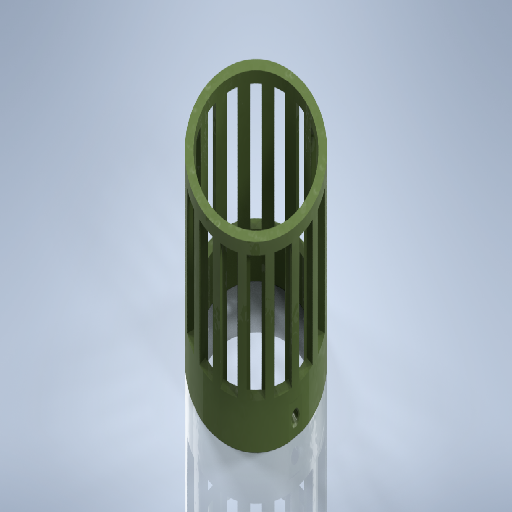
# Autodesk Inventor part: magnet_ring
Saved by Autodesk Inventor 2025 (Build 290162000, 162)
## iProperties
Created: 2026-08-03
Part Number: magnet_ring
Material: Ogólny
Document SubType Name: Modeling
Designer: zzapa
Density: 1 g/cm^3
Appearance: Ciemnooliwkowa
Author: zzapa
Autodesk Inventor part; units mm, degrees
ref_plane "YZ Plane" through (0, 0, 0) normal (1, 0, 0) x (0, 1, 0)
ref_plane "XZ Plane" through (0, 0, 0) normal (0, 1, 0) x (-1, 0, 0)
sketch "Szkic1" plane through (0, 0, 0) normal (0, 0, 1) x (1, 0, 0)
  line L0 (26.95, 18) -> (23.65, 18)
  line L1 (23.65, 18) -> (23.65, -18)
  line L2 (23.65, -18) -> (26.95, -18)
  line L3 (26.95, -18) -> (26.95, 18)
  line L4 (-5.39, 0) -> (32.34, 0) projected
  line L5 (0, -25.2) -> (0, 25.2) projected
  point P0 (0, 0)
  point P1 (23.65, 0)
  dimension "d0" = 26.95
  dimension "d1" = 3.3
  dimension "d15" = 36
  constraints: 8 end point, 2 parallel, 1 horizontal, 1 midpoint, 1 perpendicular, 1 point on line
  measures "d0" distance from line of point (0, 0) L3
  measures "d1" distance of L0.start L0.end
  measures "d15" distance of L2.end L0.start
revolve "Obrót1" add sketch "Szkic1" angle 360 about axis through (0, -10, 0) along (0, 1, 0)
sketch "Szkic2" plane through (0, 0, 0) normal (0, 1, 0) x (-1, 0, 0)
  line L0 (23.615164, -3.55) -> (26.715164, -3.55)
  line L1 (26.715164, -3.55) -> (26.715164, 3.55)
  line L2 (26.715164, 3.55) -> (23.615164, 3.55)
  line L3 (23.615164, 3.55) -> (23.615164, -3.55)
  circle A0 centre (0, 0) radius 26.95
  line L4 (37.73, 0) -> (-37.73, 0)
  line L5 (26.715164, -3.55) -> (26.95, -3.55)
  line L6 (26.95, -3.55) -> (26.95, 3.55)
  line L7 (26.95, 3.55) -> (26.715164, 3.55)
  line L8 (26.715164, 3.55) -> (26.715164, -3.55)
  line L9 (23.55207, -2.15) -> (23.615164, -2.15)
  line L10 (23.615164, -2.15) -> (23.615164, 2.15)
  line L11 (23.615164, 2.15) -> (23.55207, 2.15)
  line L12 (23.55207, 2.15) -> (23.55207, -2.15)
  circle A1 centre (0, 0) radius 23.65
  line L13 (22.582045, 7.026646) -> (22.640336, 7.050791)
  line L14 (20.936506, 10.999328) -> (22.582045, 7.026646)
  line L15 (22.640336, 7.050791) -> (20.994798, 11.023473)
  line L16 (20.459041, 12.316904) -> (23.176093, 5.75736)
  line L17 (23.176093, 5.75736) -> (26.04012, 6.943678)
  line L18 (23.323067, 13.503223) -> (20.459041, 12.316904)
  line L19 (26.04012, 6.943678) -> (26.25708, 7.033546)
  line L20 (23.540027, 13.593091) -> (23.323067, 13.503223)
  line L21 (26.04012, 6.943678) -> (23.323067, 13.503223)
  line L22 (23.323067, 13.503223) -> (26.04012, 6.943678)
  line L23 (26.25708, 7.033546) -> (23.540027, 13.593091)
  line L24 (20.994798, 11.023473) -> (20.936506, 10.999328)
  line L25 (18.174108, 15.133549) -> (18.218722, 15.178163)
  line L26 (15.133549, 18.174108) -> (18.174108, 15.133549)
  line L27 (18.218722, 15.178163) -> (15.178163, 18.218722)
  line L28 (14.188214, 19.208672) -> (19.208672, 14.188214)
  line L29 (19.208672, 14.188214) -> (21.400703, 16.380245)
  line L30 (16.380245, 21.400703) -> (14.188214, 19.208672)
  line L31 (21.400703, 16.380245) -> (21.566757, 16.546299)
  line L32 (16.546299, 21.566757) -> (16.380245, 21.400703)
  line L33 (21.400703, 16.380245) -> (16.380245, 21.400703)
  line L34 (16.380245, 21.400703) -> (21.400703, 16.380245)
  line L35 (21.566757, 16.546299) -> (16.546299, 21.566757)
  line L36 (15.178163, 18.218722) -> (15.133549, 18.174108)
  line L37 (10.999328, 20.936506) -> (11.023473, 20.994798)
  line L38 (7.026646, 22.582045) -> (10.999328, 20.936506)
  line L39 (11.023473, 20.994798) -> (7.050791, 22.640336)
  line L40 (5.75736, 23.176093) -> (12.316904, 20.459041)
  line L41 (12.316904, 20.459041) -> (13.503223, 23.323067)
  line L42 (6.943678, 26.04012) -> (5.75736, 23.176093)
  line L43 (13.503223, 23.323067) -> (13.593091, 23.540027)
  line L44 (7.033546, 26.25708) -> (6.943678, 26.04012)
  line L45 (13.503223, 23.323067) -> (6.943678, 26.04012)
  line L46 (6.943678, 26.04012) -> (13.503223, 23.323067)
  line L47 (13.593091, 23.540027) -> (7.033546, 26.25708)
  line L48 (7.050791, 22.640336) -> (7.026646, 22.582045)
  line L49 (2.15, 23.55207) -> (2.15, 23.615164)
  line L50 (-2.15, 23.55207) -> (2.15, 23.55207)
  line L51 (2.15, 23.615164) -> (-2.15, 23.615164)
  line L52 (-3.55, 23.615164) -> (3.55, 23.615164)
  line L53 (3.55, 23.615164) -> (3.55, 26.715164)
  line L54 (-3.55, 26.715164) -> (-3.55, 23.615164)
  line L55 (3.55, 26.715164) -> (3.55, 26.95)
  line L56 (-3.55, 26.95) -> (-3.55, 26.715164)
  line L57 (3.55, 26.715164) -> (-3.55, 26.715164)
  line L58 (-3.55, 26.715164) -> (3.55, 26.715164)
  line L59 (3.55, 26.95) -> (-3.55, 26.95)
  line L60 (-2.15, 23.615164) -> (-2.15, 23.55207)
  line L61 (-7.026646, 22.582045) -> (-7.050791, 22.640336)
  line L62 (-10.999328, 20.936506) -> (-7.026646, 22.582045)
  line L63 (-7.050791, 22.640336) -> (-11.023473, 20.994798)
  line L64 (-12.316904, 20.459041) -> (-5.75736, 23.176093)
  line L65 (-5.75736, 23.176093) -> (-6.943678, 26.04012)
  line L66 (-13.503223, 23.323067) -> (-12.316904, 20.459041)
  line L67 (-6.943678, 26.04012) -> (-7.033546, 26.25708)
  line L68 (-13.593091, 23.540027) -> (-13.503223, 23.323067)
  line L69 (-6.943678, 26.04012) -> (-13.503223, 23.323067)
  line L70 (-13.503223, 23.323067) -> (-6.943678, 26.04012)
  line L71 (-7.033546, 26.25708) -> (-13.593091, 23.540027)
  line L72 (-11.023473, 20.994798) -> (-10.999328, 20.936506)
  line L73 (-15.133549, 18.174108) -> (-15.178163, 18.218722)
  line L74 (-18.174108, 15.133549) -> (-15.133549, 18.174108)
  line L75 (-15.178163, 18.218722) -> (-18.218722, 15.178163)
  line L76 (-19.208672, 14.188214) -> (-14.188214, 19.208672)
  line L77 (-14.188214, 19.208672) -> (-16.380245, 21.400703)
  line L78 (-21.400703, 16.380245) -> (-19.208672, 14.188214)
  line L79 (-16.380245, 21.400703) -> (-16.546299, 21.566757)
  line L80 (-21.566757, 16.546299) -> (-21.400703, 16.380245)
  line L81 (-16.380245, 21.400703) -> (-21.400703, 16.380245)
  line L82 (-21.400703, 16.380245) -> (-16.380245, 21.400703)
  line L83 (-16.546299, 21.566757) -> (-21.566757, 16.546299)
  line L84 (-18.218722, 15.178163) -> (-18.174108, 15.133549)
  line L85 (-20.936506, 10.999328) -> (-20.994798, 11.023473)
  line L86 (-22.582045, 7.026646) -> (-20.936506, 10.999328)
  line L87 (-20.994798, 11.023473) -> (-22.640336, 7.050791)
  line L88 (-23.176093, 5.75736) -> (-20.459041, 12.316904)
  line L89 (-20.459041, 12.316904) -> (-23.323067, 13.503223)
  line L90 (-26.04012, 6.943678) -> (-23.176093, 5.75736)
  line L91 (-23.323067, 13.503223) -> (-23.540027, 13.593091)
  line L92 (-26.25708, 7.033546) -> (-26.04012, 6.943678)
  line L93 (-23.323067, 13.503223) -> (-26.04012, 6.943678)
  line L94 (-26.04012, 6.943678) -> (-23.323067, 13.503223)
  line L95 (-23.540027, 13.593091) -> (-26.25708, 7.033546)
  line L96 (-22.640336, 7.050791) -> (-22.582045, 7.026646)
  line L97 (-23.55207, 2.15) -> (-23.615164, 2.15)
  line L98 (-23.55207, -2.15) -> (-23.55207, 2.15)
  line L99 (-23.615164, 2.15) -> (-23.615164, -2.15)
  line L100 (-23.615164, -3.55) -> (-23.615164, 3.55)
  line L101 (-23.615164, 3.55) -> (-26.715164, 3.55)
  line L102 (-26.715164, -3.55) -> (-23.615164, -3.55)
  line L103 (-26.715164, 3.55) -> (-26.95, 3.55)
  line L104 (-26.95, -3.55) -> (-26.715164, -3.55)
  line L105 (-26.715164, 3.55) -> (-26.715164, -3.55)
  line L106 (-26.715164, -3.55) -> (-26.715164, 3.55)
  line L107 (-26.95, 3.55) -> (-26.95, -3.55)
  line L108 (-23.615164, -2.15) -> (-23.55207, -2.15)
  line L109 (-22.582045, -7.026646) -> (-22.640336, -7.050791)
  line L110 (-20.936506, -10.999328) -> (-22.582045, -7.026646)
  line L111 (-22.640336, -7.050791) -> (-20.994798, -11.023473)
  line L112 (-20.459041, -12.316904) -> (-23.176093, -5.75736)
  line L113 (-23.176093, -5.75736) -> (-26.04012, -6.943678)
  line L114 (-23.323067, -13.503223) -> (-20.459041, -12.316904)
  line L115 (-26.04012, -6.943678) -> (-26.25708, -7.033546)
  line L116 (-23.540027, -13.593091) -> (-23.323067, -13.503223)
  line L117 (-26.04012, -6.943678) -> (-23.323067, -13.503223)
  line L118 (-23.323067, -13.503223) -> (-26.04012, -6.943678)
  line L119 (-26.25708, -7.033546) -> (-23.540027, -13.593091)
  line L120 (-20.994798, -11.023473) -> (-20.936506, -10.999328)
  line L121 (-18.174108, -15.133549) -> (-18.218722, -15.178163)
  line L122 (-15.133549, -18.174108) -> (-18.174108, -15.133549)
  line L123 (-18.218722, -15.178163) -> (-15.178163, -18.218722)
  line L124 (-14.188214, -19.208672) -> (-19.208672, -14.188214)
  line L125 (-19.208672, -14.188214) -> (-21.400703, -16.380245)
  line L126 (-16.380245, -21.400703) -> (-14.188214, -19.208672)
  line L127 (-21.400703, -16.380245) -> (-21.566757, -16.546299)
  line L128 (-16.546299, -21.566757) -> (-16.380245, -21.400703)
  line L129 (-21.400703, -16.380245) -> (-16.380245, -21.400703)
  line L130 (-16.380245, -21.400703) -> (-21.400703, -16.380245)
  line L131 (-21.566757, -16.546299) -> (-16.546299, -21.566757)
  line L132 (-15.178163, -18.218722) -> (-15.133549, -18.174108)
  line L133 (-10.999328, -20.936506) -> (-11.023473, -20.994798)
  line L134 (-7.026646, -22.582045) -> (-10.999328, -20.936506)
  line L135 (-11.023473, -20.994798) -> (-7.050791, -22.640336)
  line L136 (-5.75736, -23.176093) -> (-12.316904, -20.459041)
  line L137 (-12.316904, -20.459041) -> (-13.503223, -23.323067)
  line L138 (-6.943678, -26.04012) -> (-5.75736, -23.176093)
  line L139 (-13.503223, -23.323067) -> (-13.593091, -23.540027)
  line L140 (-7.033546, -26.25708) -> (-6.943678, -26.04012)
  line L141 (-13.503223, -23.323067) -> (-6.943678, -26.04012)
  line L142 (-6.943678, -26.04012) -> (-13.503223, -23.323067)
  line L143 (-13.593091, -23.540027) -> (-7.033546, -26.25708)
  line L144 (-7.050791, -22.640336) -> (-7.026646, -22.582045)
  line L145 (-2.15, -23.55207) -> (-2.15, -23.615164)
  line L146 (2.15, -23.55207) -> (-2.15, -23.55207)
  line L147 (-2.15, -23.615164) -> (2.15, -23.615164)
  line L148 (3.55, -23.615164) -> (-3.55, -23.615164)
  line L149 (-3.55, -23.615164) -> (-3.55, -26.715164)
  line L150 (3.55, -26.715164) -> (3.55, -23.615164)
  line L151 (-3.55, -26.715164) -> (-3.55, -26.95)
  line L152 (3.55, -26.95) -> (3.55, -26.715164)
  line L153 (-3.55, -26.715164) -> (3.55, -26.715164)
  line L154 (3.55, -26.715164) -> (-3.55, -26.715164)
  line L155 (-3.55, -26.95) -> (3.55, -26.95)
  line L156 (2.15, -23.615164) -> (2.15, -23.55207)
  line L157 (7.026646, -22.582045) -> (7.050791, -22.640336)
  line L158 (10.999328, -20.936506) -> (7.026646, -22.582045)
  line L159 (7.050791, -22.640336) -> (11.023473, -20.994798)
  line L160 (12.316904, -20.459041) -> (5.75736, -23.176093)
  line L161 (5.75736, -23.176093) -> (6.943678, -26.04012)
  line L162 (13.503223, -23.323067) -> (12.316904, -20.459041)
  line L163 (6.943678, -26.04012) -> (7.033546, -26.25708)
  line L164 (13.593091, -23.540027) -> (13.503223, -23.323067)
  line L165 (6.943678, -26.04012) -> (13.503223, -23.323067)
  line L166 (13.503223, -23.323067) -> (6.943678, -26.04012)
  line L167 (7.033546, -26.25708) -> (13.593091, -23.540027)
  line L168 (11.023473, -20.994798) -> (10.999328, -20.936506)
  line L169 (15.133549, -18.174108) -> (15.178163, -18.218722)
  line L170 (18.174108, -15.133549) -> (15.133549, -18.174108)
  line L171 (15.178163, -18.218722) -> (18.218722, -15.178163)
  line L172 (19.208672, -14.188214) -> (14.188214, -19.208672)
  line L173 (14.188214, -19.208672) -> (16.380245, -21.400703)
  line L174 (21.400703, -16.380245) -> (19.208672, -14.188214)
  line L175 (16.380245, -21.400703) -> (16.546299, -21.566757)
  line L176 (21.566757, -16.546299) -> (21.400703, -16.380245)
  line L177 (16.380245, -21.400703) -> (21.400703, -16.380245)
  line L178 (21.400703, -16.380245) -> (16.380245, -21.400703)
  line L179 (16.546299, -21.566757) -> (21.566757, -16.546299)
  line L180 (18.218722, -15.178163) -> (18.174108, -15.133549)
  line L181 (20.936506, -10.999328) -> (20.994798, -11.023473)
  line L182 (22.582045, -7.026646) -> (20.936506, -10.999328)
  line L183 (20.994798, -11.023473) -> (22.640336, -7.050791)
  line L184 (23.176093, -5.75736) -> (20.459041, -12.316904)
  line L185 (20.459041, -12.316904) -> (23.323067, -13.503223)
  line L186 (26.04012, -6.943678) -> (23.176093, -5.75736)
  line L187 (23.323067, -13.503223) -> (23.540027, -13.593091)
  line L188 (26.25708, -7.033546) -> (26.04012, -6.943678)
  line L189 (23.323067, -13.503223) -> (26.04012, -6.943678)
  line L190 (26.04012, -6.943678) -> (23.323067, -13.503223)
  line L191 (23.540027, -13.593091) -> (26.25708, -7.033546)
  line L192 (22.640336, -7.050791) -> (22.582045, -7.026646)
  point P0 (26.715164, 0)
  point P1 (26.95, 0)
  point P2 (23.55207, 0)
  point P3 (21.759275, 9.012987)
  point P4 (24.681593, 10.223451)
  point P5 (24.898553, 10.313319)
  point P6 (16.653828, 16.653828)
  point P7 (18.890474, 18.890474)
  point P8 (19.056528, 19.056528)
  point P9 (9.012987, 21.759275)
  point P10 (10.223451, 24.681593)
  point P11 (10.313319, 24.898553)
  point P12 (0, 23.55207)
  point P13 (0, 26.715164)
  point P14 (0, 26.95)
  point P15 (-9.012987, 21.759275)
  point P16 (-10.223451, 24.681593)
  point P17 (-10.313319, 24.898553)
  point P18 (-16.653828, 16.653828)
  point P19 (-18.890474, 18.890474)
  point P20 (-19.056528, 19.056528)
  point P21 (-21.759275, 9.012987)
  point P22 (-24.681593, 10.223451)
  point P23 (-24.898553, 10.313319)
  point P24 (-23.55207, 0)
  point P25 (-26.715164, 0)
  point P26 (-26.95, 0)
  point P27 (-21.759275, -9.012987)
  point P28 (-24.681593, -10.223451)
  point P29 (-24.898553, -10.313319)
  point P30 (-16.653828, -16.653828)
  point P31 (-18.890474, -18.890474)
  point P32 (-19.056528, -19.056528)
  point P33 (-9.012987, -21.759275)
  point P34 (-10.223451, -24.681593)
  point P35 (-10.313319, -24.898553)
  point P36 (0, -23.55207)
  point P37 (0, -26.715164)
  point P38 (0, -26.95)
  point P39 (9.012987, -21.759275)
  point P40 (10.223451, -24.681593)
  point P41 (10.313319, -24.898553)
  point P42 (16.653828, -16.653828)
  point P43 (18.890474, -18.890474)
  point P44 (19.056528, -19.056528)
  point P45 (21.759275, -9.012987)
  point P46 (24.681593, -10.223451)
  point P47 (24.898553, -10.313319)
  point P48 (22.582045, 7.026646)
  point P49 (22.640336, 7.050791)
  point P50 (20.994798, 11.023473)
  point P51 (20.936506, 10.999328)
  point P52 (18.174108, 15.133549)
  point P53 (18.218722, 15.178163)
  point P54 (15.178163, 18.218722)
  point P55 (15.133549, 18.174108)
  point P56 (10.999328, 20.936506)
  point P57 (11.023473, 20.994798)
  point P58 (7.050791, 22.640336)
  point P59 (2.15, 23.55207)
  point P60 (2.15, 23.615164)
  point P61 (-2.15, 23.615164)
  point P62 (-7.026646, 22.582045)
  point P63 (-7.050791, 22.640336)
  point P64 (-11.023473, 20.994798)
  point P65 (-10.999328, 20.936506)
  point P66 (-15.133549, 18.174108)
  point P67 (-15.178163, 18.218722)
  point P68 (-18.218722, 15.178163)
  point P69 (-18.174108, 15.133549)
  point P70 (-20.936506, 10.999328)
  point P71 (-20.994798, 11.023473)
  point P72 (-22.640336, 7.050791)
  point P73 (-23.55207, 2.15)
  point P74 (-23.615164, 2.15)
  point P75 (-23.615164, -2.15)
  point P76 (-23.55207, -2.15)
  point P77 (-22.582045, -7.026646)
  point P78 (-22.640336, -7.050791)
  point P79 (-20.994798, -11.023473)
  point P80 (-20.936506, -10.999328)
  point P81 (-18.174108, -15.133549)
  point P82 (-18.218722, -15.178163)
  point P83 (-15.178163, -18.218722)
  point P84 (-15.133549, -18.174108)
  point P85 (-10.999328, -20.936506)
  point P86 (-11.023473, -20.994798)
  point P87 (-7.050791, -22.640336)
  point P88 (-2.15, -23.55207)
  point P89 (-2.15, -23.615164)
  point P90 (2.15, -23.615164)
  point P91 (2.15, -23.55207)
  point P92 (7.026646, -22.582045)
  point P93 (11.023473, -20.994798)
  point P94 (10.999328, -20.936506)
  point P95 (15.133549, -18.174108)
  point P96 (18.218722, -15.178163)
  point P97 (18.174108, -15.133549)
  point P98 (20.936506, -10.999328)
  point P99 (22.640336, -7.050791)
  point P100 (22.582045, -7.026646)
  point P101 (23.615164, -2.15)
  point P102 (23.615164, 2.15)
  dimension "d3" = 7.1
  dimension "d4" = 3.1
  dimension "d16" = 1.4
  dimension "d19" = 360
  constraints: 384 end point, 6 parallel, 3 horizontal, 3 midpoint, 3 perpendicular, 2 collinear, 2 point on circle, 2 point on line, 419 other
  measures "d3" distance of L0.end L1.end
  measures "d4" distance of L1.end L2.end
  measures "d16" distance between parallel lines of L11 L2
extrude "Pocket" cut sketch "Szkic2" along normal mid plane 30.3 contours L3 A1 L4 L1 L0 | L1 L4 A0 | A0 L6 L5 | L9 A1 L3 | L4 A1 L3 L2 L1 | L1 A0 L4 | L188 L191 A0 | L189 L185 L184 L183 A1 L186 | A0 L189 | A0 L7 L6 | A1 L12 L4 L3 | L3 L4 A1 | A1 L182 L170 L158 L146 L134 L122 L110 L98 L4 L12 | L4 L3 A1 | L191 L187 A0 | L4 L12 A1 L3 | L4 L98 A1 L86 L74 L62 L50 L38 L26 L14 L12 | L192 L183 A1 | A1 L183 L182 | L21 A0 | A0 L23 L19 | L17 L16 L15 A1 L18 L21 | A1 L11 L3 | L176 L179 A0 | L177 L173 L172 L171 A1 L174 | A0 L177 | L98 A1 L99 L4 | L4 L99 A1 L98 | A1 L183 | A1 L183 L181 | A0 L20 L23 | L179 L175 A0 | L99 A1 L4 | L4 A1 L99 | L108 L99 A1 | A1 L99 L97 | L14 A1 L15 | A1 L15 L13 | L180 L171 A1 | A1 L171 L170 | L33 A0 | A0 L35 L31 | L29 L28 L27 A1 L30 L33 | L164 L167 A0 | L165 L161 L160 L159 A1 L162 | A0 L165 | A1 L99 L100 L102 A0 L4 | L4 A0 L101 L100 L99 A1 | L110 A1 L111 | A1 L111 L109 | L96 L87 A1 | A1 L87 L86 | L15 A1 | L24 L15 A1 | A1 L171 | A1 L171 L169 | A0 L32 L35 | L167 L163 A0 | L111 A1 | A1 L111 L112 L114 L117 L113 | L120 L111 A1 | L87 L88 L90 L93 L89 A1 | A1 L87 | A1 L87 L85 | L26 A1 L27 | A1 L27 L25 | L168 L159 A1 | A1 L159 L158 | L45 A0 | A0 L47 L43 | L41 L40 L39 A1 L42 L45 | L152 L155 A0 | L153 L149 L148 L147 A1 L150 | A0 L153 | L122 A1 L123 | A1 L123 L121 | L84 L75 A1 | A1 L75 L74 | L27 A1 | L36 L27 A1 | A1 L159 | A1 L159 L157 | A0 L44 L47 | L155 L151 A0 | L92 L95 A0 | A0 L93 | L117 A0 | A0 L119 L115 | L123 A1 | A1 L123 L124 L126 L129 L125 | L132 L123 A1 | L75 L76 L78 L81 L77 A1 | A1 L75 | A1 L75 L73 | L38 A1 L39 | A1 L39 L37 | L156 L147 A1 | A1 L147 L146 | L57 A0 | A0 L59 L55 | L53 L52 L51 A1 L54 L57 | L140 L143 A0 | L141 L137 L136 L135 A1 L138 | A0 L141 | L95 L91 A0 | A0 L116 L119 | L134 A1 L135 | A1 L135 L133 | L72 L63 A1 | A1 L63 L62 | L39 A1 | L48 L39 A1 | A1 L147 | A1 L147 L145 | A0 L56 L59 | L143 L139 A0 | L80 L83 A0 | A0 L81 | L129 A0 | A0 L131 L127 | L135 A1 | L144 L135 A1 | L63 L64 L66 L69 L65 A1 | A1 L63 | A1 L63 L61 | L50 A1 L51 | A1 L51 L49 | L69 A0 | A0 L71 L67 | L128 L131 A0 | L83 L79 A0 | L60 L51 A1 | L51 A1 | A0 L68 L71
sketch "Szkic3" plane through (0, -18, 0) normal (0, -1, 0) x (1, 0, 0)
  circle A0 centre (0, 0) radius 26.95
  circle A1 centre (0, 0) radius 23.65
  circle A2 centre (0, 0) radius 23.65
  line L0 (3.55, -26.715164) -> (3.55, -23.615164)
  circle A3 centre (0, 0) radius 26.95
  constraints: 2 coincident, 1 centre point, 1 concentric, 4 other
extrude "Wyciągnięcie proste2" add sketch "Szkic3" along normal blind 8
ref_plane "Płaszczyzna konstrukcyjna3" through (-26.432163, 0, -5.257684) normal (-0.9807853, 0, -0.1950903) x (0, -1, 0)
ref_plane "Płaszczyzna konstrukcyjna2" through (-4.697348, -15.15, 23.615164) normal (-0.9807853, 0, -0.1950903) x (0, -1, 0)
sketch "Szkic5" plane through (0, -26, 0) normal (0, -1, 0) x (1, 0, 0)
  circle A0 centre (0, 0) radius 26.95
  line L0 (-17.686376, -49.225728) -> (-35.630211, 40.984024)
  line L1 (-27.021778, -2.293489) -> (-25.842548, -8.22188)
  line L2 (-25.842548, -8.22188) -> (-25.675815, -8.188714)
  line L3 (-25.675815, -8.188714) -> (-26.855045, -2.260323)
  line L4 (-26.855045, -2.260323) -> (-27.021778, -2.293489)
  line L5 (0, 0) -> (-38.832746, -7.724313)
  point P0 (-26.432163, -5.257684)
  dimension "d30" = 0.17
  constraints: 10 end point, 3 point on line, 2 parallel, 2 perpendicular, 1 midpoint, 2 other
  measures "d30" distance between parallel lines of L0 L3
sketch "Szkic5 outline for Wyciągnięcie proste4" plane through (0, -26, 0) normal (0, -1, 0) x (1, 0, 0)
  line L0 (-25.675815, -8.188714) -> (-26.855045, -2.260323)
  line L1 (-25.842548, -8.22188) -> (-25.675815, -8.188714)
  line L2 (-27.021778, -2.293489) -> (-25.842548, -8.22188)
  line L3 (-26.855045, -2.260323) -> (-27.021778, -2.293489)
extrude "Wyciągnięcie proste4" cut sketch "Szkic5 outline for Wyciągnięcie proste4" against normal blind 8
mirror "Odbij1" about plane through (-4.697348, -15.15, 23.615164) normal (-0.9807853, 0, -0.1950903) of "Wyciągnięcie proste4"
sketch "Szkic6" plane through (-26.855045, -26, -2.260323) normal (-0.9807853, 0, -0.1950903) x (-0.1950903, 0, 0.9807853)
  line L0 (0, 8) -> (-6.044535, 8)
  line L1 (0, 0) -> (-6.044535, 0)
  line L2 (-3.022267, 8) -> (-3.022267, 0)
  line L3 (20.627733, 0) -> (-26.672267, 0)
  point P0 (-3.022267, 26)
  point P1 (-3.022267, 4)
  dimension "d31" = 4
  constraints: 3 midpoint, 2 end point
  measures "d31" distance from line of L1 point (-3.022, 4)
hole "Otwór1" at (-26.26543, -22, -5.224519) direction (0.9807853, 0, 0.1950903) diameter 2.9 end through all
chamfer "Faza1" distance 0.5 angle 45 2 edges at (-25.9825, -22, -6.6467) (26.5483, -22, 3.8024)
sketch "Szkic7" plane through (-26.855045, -26, -2.260323) normal (-0.9807853, 0, -0.1950903) x (-0.1950903, 0, 0.9807853)
  circle A0 centre (-3.022267, 4) radius 1.45
  line L0 (-3.022267, 4) -> (-3.022267, 8)
  line L1 (0, 0) -> (-6.044535, 0)
  line L2 (0, 8) -> (-6.044535, 8)
  line L3 (-3.022267, 5.674316) -> (-3.747267, 5.255737)
  line L4 (-3.022267, 5.674316) -> (-2.297267, 5.255737)
  point P0 (-3.022267, 26)
  point P1 (-2.297267, 5.255737)
  dimension "d45" = 120
  constraints: 6 end point, 1 midpoint, 1 point on line, 1 symmetric about line, 1 vertical, 3 other
  measures "d45" angle of L3 L4
extrude "Wyciągnięcie proste5" cut sketch "Szkic7" against normal through all contours A0 L0 L4 | L3 L0 A0
equation "\"d0\" = magnet_ring_r"
equation "\"d1\" = magnet_ring_d"
equation "\"d15\" = magnet_ring_h"
equation "\"d3\" = magnet_ring_pocket_mag_size_x"
equation "\"d4\" = magnet_ring_pocket_mag_size_y"
equation "\"d16\" = magnet_ring_pocket_radial_cut"
equation "\"d9\" = 3 * magnet_ring_pocket_mag_size_z"
equation "\"d21\" = magnet_ring_insert_part_lengthen"
equation "\"d30\" = magnet_ring_insert_part_axial_flat_cut"
equation "\"d31\" = magnet_ring_insert_pos"
equation "\"d32\" = insert_m2_d"
equation "\"d42\" = insert_m2_corner"
equation "\"stator_r_out\" = 30.15"
equation "\"stator_out_d\" = 3.2"
equation "\"stator_h\" = 45"
equation "\"mag_size_x\" = 7"
equation "\"mag_size_y\" = 3"
equation "\"mag_corner_r\" = 0.4"
equation "\"magnet_ring_r\" = 26.95"
equation "\"magnet_ring_d\" = 3.3"
equation "\"magnet_ring_pocket_mag_size_y\" = 3.1"
equation "\"magnet_ring_pocket_mag_size_x\" = 7.1"
equation "\"magnet_ring_pocket_mag_size_z\" = 10.1"
equation "\"magnet_ring_mag_count\" = 16"
equation "\"magnet_ring_h\" = 36"
equation "\"magnet_ring_pocket_radial_cut\" = 1.4"
equation "\"casing_d\" = 3"
equation "\"casing_r_in\" = 30.15"
equation "\"rotor_core_r\" = 14.97"
equation "\"coil_groove_ang\" = 18"
equation "\"rotor_out_r\" = 22.5"
equation "\"rotor_coil_groove_in_r\" = 17"
equation "\"rotor_coil_groove_ang\" = 18deg"
equation "\"rotor_coil_groove_in_correction_r\" = 18"
equation "\"rotor_plastic_h\" = 32"
equation "\"rotor_teeth_d\" = 1.5"
equation "\"shaft_d\" = 8"
equation "\"insert25m_d\" = 2.9"
equation "\"insert25m_corner\" = 0.5"
equation "\"insert25m_h\" = 7"
equation "\"rotor_plastic_insert_r\" = 37"
equation "\"shaft_lock_1_d\" = 8.1"
equation "\"shaf_lock_1_D\" = 32"
equation "\"shaft_lock_1_D\" = 44"
equation "\"shaft_lock_1_h1\" = 3.5"
equation "\"shaft_lock_1_insert_part_h\" = 8"
equation "\"shaft_lock_1_corner\" = 2"
equation "\"shaft_lock_1_insert_part_a\" = 18"
equation "\"shaft_lock_2_h1\" = 3.5"
equation "\"shaft_lock_2_d\" = 8.1"
equation "\"shaft_lock_2_insert_part_a\" = 18"
equation "\"shaft_lock_2_D\" = 44"
equation "\"shaft_lock_2_corner\" = 2"
equation "\"shaft_lock_2_insert_part_h\" = 7"
equation "\"shaft_lock_2_rotor_insert_grove_d_in\" = 36"
equation "\"shaft_lock_2_rotor_insert_grove_width_out\" = 5.5"
equation "\"shaft_lock_2_rotor_insert_grove_width_in\" = 7.6"
equation "\"shaft_lock_2_rotor_insert_r\" = 37"
equation "\"shaft_lock_2_rotor_insert_screw_d\" = 2.6"
equation "\"insert25m_pocket_d\" = 2.6"
equation "\"insert25m_pocket_D\" = 4.5"
equation "\"insert25m_pocket_nut_h\" = 1.5"
equation "\"insert_m2_pocket_d\" = 2.6"
equation "\"insert_m2_h\" = 7"
equation "\"insert_m2_d\" = 2.9"
equation "\"insert_m2_corner\" = 0.5"
equation "\"insert_m2_pocket_D\" = 4.5"
equation "\"insert_m2_pocket_nut_h\" = 1.5"
equation "\"shaft_lock_1_insert_part_corner\" = 6"
equation "\"shaft_lock_1_insert_part_pos\" = 4"
equation "\"shaft_lock_1_rotor_insert_grove_width_in\" = 7.6"
equation "\"shaft_lock_1_rotor_insert_r\" = 37"
equation "\"shaft_lock_1_rotor_insert_grove_d_in\" = 36"
equation "\"shaft_lock_1_rotor_insert_grove_width_out\" = 5.5"
equation "\"shaft_lock_1_shaft_insert_axial_cut_out_width\" = 12"
equation "\"shaft_lock_1_shaft_insert_axial_cut_in_width\" = 5.4"
equation "\"shaft_lock_1_shaft_insert_corner\" = 2"
equation "\"shaft_lock_1_shaft_insert_corner_finish\" = 0.5"
equation "\"shaft_lock_1_shaft_insert_pos\" = 2.5"
equation "\"shaft_lock_2_shaft_insert_corner\" = 2"
equation "\"shaft_lock_2_shaft_insert_pos\" = 2.5"
equation "\"shaft_lock_2_shaft_insert_axial_cut_in_width\" = 5.4"
equation "\"shaft_lock_2_shaft_insert_axial_cut_out_width\" = 12"
equation "\"shaft_lock_2_shaft_insert_corner_finish\" = 0.5"
equation "\"commutator_plate_D\" = 22"
equation "\"commutator_plastic_d\" = 1"
equation "\"commutator_plastic_h\" = 17"
equation "\"commutator_plate_ang\" = 55deg"
equation "\"commutator_plate_d\" = 1"
equation "\"commutator_plate_h\" = 17"
equation "\"commutator_plastic_shaft_d\" = 8.1"
equation "\"commutator_plastic_insert_cut_deepness\" = 0.5"
equation "\"commutator_plastic_insert_cut_length\" = 6"
equation "\"commutator_plastic_insert_pos\" = 3"
equation "\"commutator_plate_insert_pos\" = 3"
equation "\"casing_lock_hole_r\" = 14.25"
equation "\"casing_lock_h\" = 8"
equation "\"casing_stator_fix_r\" = 23"
equation "\"casing_stator_fix_h\" = 6"
equation "\"magnet_ring_insert_part_lengthen\" = 8"
equation "\"casing_sidebar_length\" = 3"
equation "\"casing_vent_hole_length\" = 4"
equation "\"casing_vent_hole_width\" = 6"
equation "\"sleeve_cup_r\" = 22"
equation "\"sleeve_cup_h\" = 4.5"
equation "\"sleeve_h\" = 7"
equation "\"sleeve_d\" = 3"
equation "\"sleeve_in_r\" = 11.1"
equation "\"casing_head_insert_r\" = 19"
equation "\"sleeve_head_insert_r\" = 19"
equation "\"magnet_ring_insert_part_radius_cut\" = 0.17"
equation "\"magnet_ring_insert_part_axial_flat_cut\" = 0.17"
equation "\"magnet_ring_insert_pos\" = 4"
equation "\"casing_radial_stator_insert_pos\" = 18.1"
equation "\"stator_radial_screw_d\" = 4"
equation "\"stator_radial_screw_pos\" = 4"
equation "\"rotor_sleeve_out_D\" = 10.5"
equation "\"rotor_sleeve_in_D\" = 8.15"
equation "\"rotor_sleeve_h\" = 32"
equation "\"carbon_brush_batt_h\" = 8"
equation "\"carbon_brush_batt_d\" = 4"
equation "\"brush_cart_outer_holder_width\" = 5.5"
equation "\"brush_cart_outer_holder_arc_r\" = 33.15"
equation "\"brush_cart_outer_holder_arc_pos\" = 1.5"
equation "\"casing_cart_hole_corner\" = 1"
equation "\"casing_cart_hole_width\" = 2.6"
equation "\"casing_cart_hole_ang\" = 90deg"
equation "\"brush_holder_batt_arc_r\" = 30.15"
equation "\"brush_holder_batt_width\" = 16"
equation "\"brush_holder_batt_insert_flat_depth\" = 6"
equation "\"brush_holder_batt_insert_flat_length\" = 6"
equation "\"brush_holder_batt_insert_flat_length_1\" = 2"
